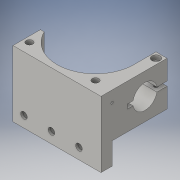
# Autodesk Inventor part: Galvomount-22mm-diameter-Thorlabs-Left
Saved by Autodesk Inventor 2016 (Build 200138000, 138)
## iProperties
Created: 2016-08-10
Part Number: Galvomount-22mm-diameter-Thorlabs-Left
Material: Generic
Document SubType Name: Modeling
Designer: voigt
Density: 1 g/cm^3
Appearance: Default
Author: voigt
Autodesk Inventor part; units mm, degrees
note: some values were not read from the file. Chosen so that the rebuilt part matches the saved one: direction of "Hole5".
ref_plane "YZ Plane" through (0, 0, 0) normal (1, 0, 0) x (0, 1, 0)
ref_plane "XZ Plane" through (0, 0, 0) normal (0, 1, 0) x (-1, 0, 0)
ref_plane "XY Plane" through (0, 0, 0) normal (0, 0, 1) x (1, 0, 0)
sketch "Sketch1" plane through (0, 0, 0) normal (0, 0, 1) x (1, 0, 0)
  line L0 (0, 32) -> (0, -52) construction
  line L1 (-59.4, 0) -> (76.4, 0) construction
  line L2 (-40, 20) -> (57, 20)
  line L3 (57, 20) -> (57, -40)
  line L4 (57, -40) -> (-40, -40)
  line L5 (-40, -40) -> (-40, 20)
  point P0 (0, 0)
  dimension "d0" = 20
  dimension "d1" = 40
  dimension "d2" = 40
  dimension "d3" = 57
  constraints: 8 end point, 2 parallel, 1 horizontal, 1 perpendicular
  measures "d0" distance between parallel lines of L1 L2
  measures "d1" distance between parallel lines of L4 L1
  measures "d2" distance between parallel lines of L5 L0
  measures "d3" distance between parallel lines of L0 L3
extrude "Extrusion1" add sketch "Sketch1" against normal blind 40
sketch "Sketch2" plane through (0, 0, 0) normal (0, 0, 1) x (1, 0, 0)
  line L0 (-40, 20) -> (57, 20) construction
  line L1 (-40, -40) -> (-40, 20) construction
  line L2 (57, -40) -> (-40, -40) construction
  line L3 (57, 20) -> (57, -40) construction
  line L4 (0, 98) -> (0, -63) construction
  line L5 (-59.4, 0) -> (76.4, 0) construction
  line L6 (0, 40) -> (0, 0) construction
  line L7 (-40, 20) -> (57, 20) projected
  line L8 (-35, 40) -> (-35, 0)
  line L9 (35, 0) -> (35, 40)
  arc A0 (35, 40) -> (-35, 40) centre (0, 40) ccw
  arc A1 (-35, 0) -> (35, 0) centre (0, 0) ccw
  point P0 (0, 20)
  dimension "d6" = 70
  constraints: 8 end point, 4 point on circle, 4 tangent, 2 centre point, 2 point on line, 1 midpoint, 1 parallel, 1 perpendicular
  measures "d6" diameter of A1
extrude "Extrusion2" cut sketch "Sketch2" against normal blind 22
sketch "Sketch3" plane through (57, -40, 0) normal (1, 0, 0) x (0, 0, -1)
  line L0 (0, 60) -> (0, 0) construction
  line L1 (0, 0) -> (40, 0) construction
  line L2 (40, 60) -> (40, 0) construction
  line L3 (0, 60) -> (40, 60) construction
  line L4 (0, 40) -> (40, 40) construction
  line L5 (40, 0) -> (40, 60) construction
  line L6 (0, 60) -> (40, 60) construction
  line L7 (20, 60) -> (20, 0) construction
  circle A0 centre (20, 40) radius 11
  dimension "d9" = 22
  constraints: 4 end point, 3 midpoint, 2 point on line, 1 centre point, 1 perpendicular
  measures "d9" diameter of A0
extrude "Extrusion3" cut sketch "Sketch3" against normal blind 65
sketch "Sketch4" plane through (57, -40, 0) normal (1, 0, 0) x (0, 0, -1)
  circle A0 centre (20, 40) radius 11 construction
  line L0 (0, 60) -> (0, 0) construction
  line L1 (0, 0) -> (40, 0) construction
  line L2 (40, 60) -> (40, 0) construction
  line L3 (0, 60) -> (40, 60) construction
  line L4 (0, 60) -> (40, 60) construction
  line L5 (20, 60) -> (20, 0) construction
  line L6 (0, 0) -> (40, 0) construction
  line L7 (0, 40) -> (40, 40) construction
  line L8 (18, 60) -> (22, 60)
  line L9 (22, 60) -> (22, 24)
  line L10 (22, 24) -> (18, 24)
  line L11 (18, 24) -> (18, 60)
  dimension "d12" = 16
  dimension "d13" = 4
  constraints: 12 end point, 2 midpoint, 2 parallel, 2 perpendicular, 2 point on line, 1 horizontal, 1 other
  measures "d12" distance between parallel lines of L7 L10
  measures "d13" distance between parallel lines of L11 L9
extrude "Extrusion4" cut sketch "Sketch4" against normal blind 70
sketch "Sketch6" plane through (0, 0, 0) normal (0, 0, 1) x (1, 0, 0)
  line L0 (0, 44) -> (0, -54) construction
  line L1 (-59.4, 0) -> (76.4, 0) construction
  line L2 (-30, 30) -> (30, 30) construction
  line L3 (30, 30) -> (30, -30) construction
  line L4 (30, -30) -> (-30, -30) construction
  line L5 (-30, -30) -> (-30, 30) construction
  point P0 (0, 0)
  dimension "d19" = 60
  dimension "d20" = 60
  constraints: 8 end point, 2 coincident, 2 parallel, 1 horizontal, 1 perpendicular, 2 other
  measures "d19" distance of L2.start L2.end
  measures "d20" distance of L4.end L2.start
hole "Hole1" at (-30, -30, 0) at (30, -30, 0) direction (0, 0, -1) diameter 6 depth 30 tip angle 118
sketch "Sketch7" plane through (0, 0, -40) normal (0, 0, -1) x (-1, 0, 0)
  line L0 (40, 20) -> (-57, 20) construction
  line L1 (-57, 20) -> (-57, -40) construction
  line L2 (-57, -40) -> (40, -40) construction
  line L3 (40, -40) -> (40, 20) construction
  line L4 (0, -52) -> (0, 32) construction
  line L5 (-76.4, 0) -> (59.4, 0) construction
  line L6 (40, 20) -> (-15, 20)
  line L7 (-15, 20) -> (-15, -15)
  line L8 (-15, -15) -> (40, -15)
  line L9 (40, -15) -> (40, 20)
  point P0 (0, 0)
  dimension "d28" = 15
  dimension "d29" = 15
  constraints: 8 end point, 2 parallel, 1 horizontal, 1 perpendicular
  measures "d28" distance between parallel lines of L4 L7
  measures "d29" distance between parallel lines of L8 L5
extrude "Extrusion6" cut sketch "Sketch7" against normal up to next
fillet "Fillet1" radius 15 1 edges at (15, -15, -31)
sketch "Sketch8" plane through (0, 0, -40) normal (0, 0, -1) x (-1, 0, 0)
  line L0 (40, -15) -> (0, -15) construction
  arc A0 (-15, 0) -> (0, -15) centre (0, 0) ccw construction
  line L1 (-15, 0) -> (-15, 20) construction
  line L2 (-15, 20) -> (-57, 20) construction
  line L3 (-57, 20) -> (-57, -40) construction
  line L4 (-57, -40) -> (40, -40) construction
  line L5 (40, -40) -> (40, -15) construction
  line L6 (-57, 20) -> (-57, -40) projected
  line L7 (40, -40) -> (-57, -40)
  line L8 (-57, -40) -> (-57, -30)
  line L9 (-57, -30) -> (40, -30)
  line L10 (40, -30) -> (40, -40)
  point P0 (0, 0)
  dimension "d33" = 10
  constraints: 8 end point, 2 parallel, 1 horizontal, 1 perpendicular, 1 point on line
  measures "d33" distance of L7.end L8.end
extrude "Extrusion7" add sketch "Sketch8" along normal blind 20
sketch "Sketch13" plane through (-40, -30, -40) normal (0, 1, 0) x (1, 0, 0)
  line L0 (40, 32) -> (40, -52) construction
  line L1 (97, 0) -> (0, 0) construction
  line L2 (97, 0) -> (97, 20) construction
  line L3 (0, 20) -> (97, 20) construction
  line L4 (0, 0) -> (0, 20) construction
  line L5 (97, -40) -> (97, 20) construction
  line L6 (97, 10) -> (0, 10) construction
  point P0 (40, -40)
  point P1 (40, 10)
  point P2 (65, 10)
  point P3 (90, 10)
  point P4 (15, 10)
  dimension "d60" = 25
  dimension "d61" = 25
  dimension "d62" = 25
  constraints: 6 point on line, 2 end point, 1 midpoint
  measures "d60" distance of point (40, 10) point (65, 10)
  measures "d61" distance of point (65, 10) point (90, 10)
  measures "d62" distance of point (40, 10) point (15, 10)
hole "Hole4" at (0, -30, -50) at (25, -30, -50) at (50, -30, -50) at (-25, -30, -50) direction (0, -1, 0) diameter 6 end through all counterbore diameter 10 counterbore depth 8
sketch "Sketch14" plane through (0, 0, 0) normal (0, 0, 1) x (1, 0, 0)
  line L0 (-31.6228, -15) -> (-40, -15) construction
  line L1 (-40, -40) -> (-40, -15) construction
  line L2 (57, -40) -> (-40, -40) construction
  line L3 (57, 20) -> (57, -40) construction
  line L4 (35, 20) -> (57, 20) construction
  line L5 (35, 20) -> (35, 0) construction
  arc A0 (-31.6228, -15) -> (35, 0) centre (0, 0) ccw construction
  circle A1 centre (30, -30) radius 3 construction
  circle A2 centre (-30, -30) radius 3 construction
  line L6 (57, 15) -> (35, 15) construction
  point P0 (40, 15)
  dimension "d70" = 5
  dimension "d106" = 5
  constraints: 3 point on line, 2 end point, 1 perpendicular
  measures "d70" distance between parallel lines of L4 L6
  measures "d106" distance from line of L5 point (40, 15)
hole "Hole5" at (40, 15, 0) direction (0, 0, -1) diameter 4 end up to surface counterbore diameter 7.5 counterbore depth 4
sketch "Sketch15" plane through (0, 0, -22) normal (0, 0, 1) x (1, 0, 0)
  circle A0 centre (40, 15) radius 2 construction
  point P0 (0, 0)
  constraints: 1 coincident
hole "Hole6" at (40, 15, -22) direction (0, 0, -1) diameter 3.242 end through all thread size "M4x0.7" class "6H" standard "ANSI Metric M Profile"
sketch "Sketch16" plane through (-40, -40, 0) normal (-1, 0, 0) x (0, 0, 1)
  line L0 (0, 25) -> (-40, 25) construction
  line L1 (-40, 10) -> (-40, 25) construction
  line L2 (-40, 10) -> (-60, 10) construction
  line L3 (-60, 0) -> (-60, 10) construction
  line L4 (0, 0) -> (-60, 0) construction
  line L5 (0, 0) -> (0, 25) construction
  line L6 (0, 13) -> (0, 7) construction
  line L7 (-30, 7) -> (-30, 13) construction
  line L8 (-30, 10) -> (0, 10) construction
  point P0 (0, 40)
  point P1 (-10, 10)
  dimension "d86" = 10
  constraints: 2 end point, 2 midpoint, 1 point on line
  measures "d86" distance from line of L5 point (-10, 10)
hole "Hole7" at (-40, -30, -10) direction (1, 0, 0) diameter 2.156 depth 8.865 tip angle 118 thread size "4-40 UNC" class "2B" standard "ANSI Unified Screw Threads"
sketch "Sketch18" plane through (-40, -40, 0) normal (-1, 0, 0) x (0, 0, 1)
  circle A0 centre (-10, 10) radius 1.078 projected
  line L0 (0, 25) -> (-40, 25) projected
  line L1 (-40, 10) -> (-40, 25) projected
  line L2 (-40, 10) -> (-60, 10) projected
  line L3 (-60, 0) -> (-60, 10) projected
  line L4 (0, 0) -> (-60, 0) projected
  line L5 (0, 0) -> (0, 25) projected
  point P0 (0, 40)
extrude "Extrusion10" cut sketch "Sketch18" against normal blind 5
sketch "Sketch19" plane through (57, -40, 0) normal (1, 0, 0) x (0, 0, -1)
  line L0 (18, 50.8167) -> (18, 60) projected
  line L1 (0, 60) -> (18, 60) projected
  line L2 (0, 60) -> (0, 0) projected
  line L3 (0, 0) -> (60, 0) projected
  line L4 (60, 10) -> (60, 0) projected
  line L5 (40, 10) -> (60, 10) projected
  line L6 (40, 60) -> (40, 10) projected
  line L7 (22, 60) -> (40, 60) projected
  line L8 (22, 60) -> (22, 50.8167) projected
  arc A0 (22, 29.1833) -> (22, 50.8167) centre (20, 40) ccw projected
  line L9 (22, 29.1833) -> (22, 24) projected
  line L10 (22, 24) -> (18, 24) projected
  line L11 (18, 24) -> (18, 29.1833) projected
  arc A1 (18, 50.8167) -> (18, 29.1833) centre (20, 40) ccw projected
  point P0 (0, 40)
extrude "Extrusion11" cut sketch "Sketch19" against normal blind 12
sketch "Sketch20" plane through (45, -40, 0) normal (1, 0, 0) x (0, 0, -1)
  line L0 (18, 60) -> (18, 50.8167) construction
  line L1 (0, 60) -> (18, 60) construction
  line L2 (0, 0) -> (0, 60) construction
  line L3 (60, 0) -> (0, 0) construction
  line L4 (60, 10) -> (60, 0) construction
  line L5 (40, 10) -> (60, 10) construction
  line L6 (40, 60) -> (40, 10) construction
  line L7 (22, 60) -> (40, 60) construction
  line L8 (22, 50.8167) -> (22, 60) construction
  arc A0 (22, 29.1833) -> (22, 50.8167) centre (20, 40) ccw construction
  line L9 (22, 24) -> (22, 29.1833) construction
  line L10 (18, 24) -> (22, 24) construction
  line L11 (18, 29.1833) -> (18, 24) construction
  arc A1 (18, 50.8167) -> (18, 29.1833) centre (20, 40) ccw construction
  line L12 (0, 7) -> (0, 13) construction
  line L13 (30, 13) -> (30, 7) construction
  circle A2 centre (10, 10) radius 1.078 construction
  point P0 (0, 40)
  constraints: 1 coincident
hole "Hole9" at (45, -30, -10) direction (-1, 0, 0) diameter 2.156 depth 15 tip angle 118 thread size "4-40 UNC" class "2B" standard "ANSI Unified Screw Threads"
body "Solid1"
